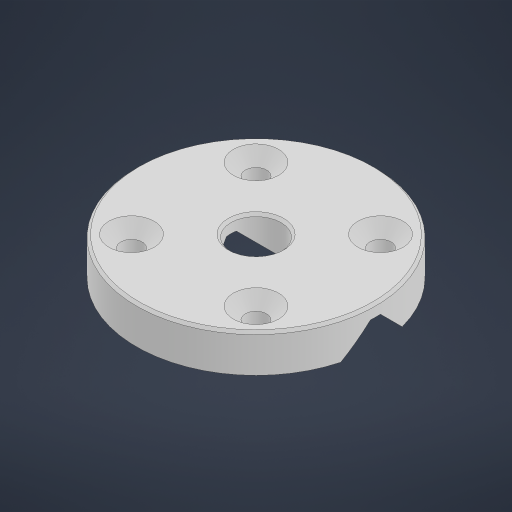
# Autodesk Inventor part: HM1_FIXT1-002
Saved by Autodesk Inventor 2024.3 (Build 283343000, 343)
## iProperties
Created: 2024-08-19
Part Number: HM1_FIXT1-002
Material: Generic
Document SubType Name: Modeling
Designer: fablabadmin
Density: 1 g/cm^3
Appearance: Default
Author: fablabadmin
Autodesk Inventor part; units mm, degrees
ref_plane "YZ Plane" through (0, 0, 0) normal (1, 0, 0) x (0, 1, 0)
ref_plane "XZ Plane" through (0, 0, 0) normal (0, 1, 0) x (-1, 0, 0)
ref_plane "XY Plane" through (0, 0, 0) normal (0, 0, 1) x (1, 0, 0)
sketch "Sketch1" plane through (0, 0, 0) normal (0, 1, 0) x (-1, 0, 0)
  circle A0 centre (0, 0) radius 47.5
  circle A1 centre (0, 0) radius 10
  circle A2 centre (0, 0) radius 35 construction
  line L0 (-24.7487, 24.7487) -> (24.7487, 24.7487) construction
  line L1 (24.7487, 24.7487) -> (24.7487, -24.7487) construction
  line L2 (24.7487, -24.7487) -> (-24.7487, -24.7487) construction
  line L3 (-24.7487, -24.7487) -> (-24.7487, 24.7487) construction
  line L4 (-24.7487, 24.7487) -> (24.7487, -24.7487) construction
  line L5 (24.7487, 24.7487) -> (-24.7487, -24.7487) construction
  dimension "d0" = 95
  dimension "d1" = 20
  dimension "d2" = 12.5
  constraints: 12 end point, 7 coincident, 2 centre point, 2 midpoint, 2 parallel, 2 perpendicular, 1 horizontal, 3 other
  measures "d0" diameter of A0
  measures "d1" diameter of A1
extrude "Extrusion1" add sketch "Sketch1" against normal blind 15
hole "Hole1" at (-24.7487, 0, -24.7487) at (24.7487, 0, -24.7487) at (24.7487, 0, 24.7487) at (-24.7487, 0, 24.7487) direction (0, -1, 0) diameter 8.5 end through all countersink diameter 18 countersink angle 90 clearance for "Countersunk Flat Head Screw ISO 2009/7046" size "M8" standard "ISO"
sketch "Sketch2" plane through (0, 0, 0) normal (1, 0, 0) x (0, 1, 0)
  line L0 (-15, 47.5) -> (-15, -47.5) projected
  line L1 (0, -47.5) -> (0, 47.5) construction
  line L2 (0, 47.5) -> (-15, 47.5) construction
  line L3 (0, -47.5) -> (-15, -47.5) construction
  line L4 (-46.8, 0) -> (7.8, 0) construction
  circle A0 centre (-24, 0) radius 15 construction
  line L5 (-15, 12.2132) -> (-4.7868, 2)
  line L6 (-4.7868, 2) -> (-4.7868, -2)
  line L7 (-4.7868, -2) -> (-15, -12.2132)
  point P0 (0, 0)
  point P1 (-4.7868, 0)
  dimension "d12" = 30
  dimension "d13" = 6
  dimension "d14" = 45
  dimension "d15" = 4
  constraints: 6 end point, 4 point on line, 1 centre point, 1 midpoint, 1 perpendicular, 1 tangent, 1 vertical
  measures "d12" diameter of A0
  measures "d13" distance edge to line of A0 L0
  measures "d14" angle of L0 L5
  measures "d15" distance of L5.end L6.end
extrude "Extrusion2" cut sketch "Sketch2" along normal through all both and the other way through all
chamfer "Chamfer1" distance 1 angle 45 2 edges at (10, 0, 0) (47.5, 0, 0)
chamfer "Chamfer3" distance 0.5 angle 45 4 edges at (24.7487, -15, 20.4987) (24.7487, -15, -28.9987) (-24.7487, -15, -28.9987) (-24.7487, -15, 20.4987)
sketch "Sketch3" plane through (45.903, -15, 12.2132) normal (0, -0.7071068, -0.7071068) x (-1, 0, 0)
  ellipse E0 centre (45.903, 17.2721) end of major axis (45.903, 3.1299) minor radius 10 (36.1051, 14.4437) -> (55.701, 14.4437) ccw construction
  line L0 (-1.5549, 14.4437) -> (36.1051, 14.4437) construction
  ellipse E1 centre (45.903, 17.2721) end of major axis (45.903, 84.4472) minor radius 47.5 (-1.5549, 14.4437) -> (0, 0) ccw construction
  line L1 (91.806, 0) -> (0, 0) construction
  ellipse E2 centre (45.903, 17.2721) end of major axis (45.903, 84.4472) minor radius 47.5 (91.806, 0) -> (93.3609, 14.4437) ccw construction
  line L2 (55.701, 14.4437) -> (93.3609, 14.4437) construction
  line L3 (92.6036, 5) -> (-0.7976, 5)
  line L4 (93.1239, 10) -> (-1.3178, 10)
  line L5 (-1.5549, 14.4437) -> (93.3609, 14.4437)
  point P0 (45.903, 19.2426)
  dimension "d27" = 5
  dimension "d30" = 5
  dimension "d31" = 4.4436
  constraints: 6 end point, 1 collinear, 1 parallel, 7 other
  measures "d27" distance between parallel lines of L1 L3
  measures "d30" distance between parallel lines of L4 L3
  measures "d31" distance between parallel lines of L2 L4
sketch "Sketch4" plane through (-45.903, -15, -12.2132) normal (0, -0.7071068, 0.7071068) x (1, 0, 0)
  ellipse E0 centre (45.903, 17.2721) end of major axis (45.903, -49.9031) minor radius 47.5 (-1.5549, 14.4437) -> (0, 0) ccw construction
  ellipse E1 centre (45.903, 17.2721) end of major axis (45.903, -49.9031) minor radius 47.5 (91.806, 0) -> (93.3609, 14.4437) ccw construction
  line L0 (92.6036, 5) -> (-0.7976, 5)
  line L1 (91.806, 0) -> (0, 0) construction
  line L2 (93.3609, 14.4437) -> (-1.5549, 14.4437)
  line L3 (-1.3178, 10) -> (93.1239, 10)
  point P0 (45.903, 19.2426)
  dimension "d29" = 5
  dimension "d32" = 5
  constraints: 6 end point, 3 horizontal, 6 other
  measures "d29" distance between parallel lines of L1 L0
  measures "d32" distance between parallel lines of L0 L3
equation "\"d30\" = d27"
equation "\"d29\" = d27"
equation "\"d32\" = d27"
body "Solid1"
